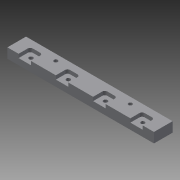
# Autodesk Inventor part: brush rack holder
Saved by Autodesk Inventor 2013 SP2 (Build 170200200, 200)
## iProperties
Created: 2017-05-30
Part Number: brush rack holder
Material: Generic
Document SubType Name: Modeling
Designer: Herman de Vries
Density: 1 g/cm^3
Author: Herman de Vries
Autodesk Inventor part; units mm, degrees
ref_plane "YZ Plane" through (0, 0, 0) normal (1, 0, 0) x (0, 1, 0)
ref_plane "XZ Plane" through (0, 0, 0) normal (0, 1, 0) x (-1, 0, 0)
ref_plane "XY Plane" through (0, 0, 0) normal (0, 0, 1) x (1, 0, 0)
sketch "Sketch1" plane through (0, 0, 0) normal (0, 0, 1) x (1, 0, 0)
  line L0 (0, 0) -> (118, 0)
  line L1 (118, 0) -> (118, 15)
  line L2 (118, 15) -> (0, 15)
  line L3 (0, 15) -> (0, 0)
  dimension "d0" = 118
  dimension "d1" = 15
  constraints: 8 end point, 2 parallel, 1 horizontal, 1 perpendicular
  measures "d0" distance of L2.end L1.end
  measures "d1" distance of L1.end L0.end
extrude "Extrusion1" add sketch "Sketch1" along normal blind 8
sketch "Sketch2" plane through (0, 0, 8) normal (0, 0, 1) x (1, 0, 0)
  circle A0 centre (14, 5) radius 1.6
  circle A1 centre (44, 5) radius 1.6
  circle A2 centre (74, 5) radius 1.6
  line L0 (0, 15) -> (0, 0) projected
  line L1 (118, 0) -> (118, 15) projected
  line L2 (0, 0) -> (118, 0) projected
  circle A3 centre (104, 5) radius 1.5
  line L3 (118, 15) -> (0, 15) projected
  circle A4 centre (29, 10) radius 1.5
  circle A5 centre (89, 10) radius 1.5
  point P0 (59, 0)
  dimension "d4" = 3.2
  dimension "d5" = 3.2
  dimension "d6" = 3.2
  dimension "d11" = 5
  dimension "d14" = 3
  dimension "d15" = 30
  dimension "d16" = 30
  dimension "d17" = 30
  dimension "d18" = 14
  dimension "d19" = 14
  dimension "d20" = 3
  dimension "d21" = 3
  dimension "d22" = 5
  dimension "d23" = 29
  dimension "d24" = 29
  constraints: 6 centre point, 4 horizontal alignment, 1 midpoint
  measures "d4" diameter of A0
  measures "d5" diameter of A1
  measures "d6" diameter of A2
  measures "d11" vertical distance of L0.end A0.centre
  measures "d14" diameter of A3
  measures "d15" distance of A0.centre A1.centre
  measures "d16" distance of A1.centre A2.centre
  measures "d17" distance of A2.centre A3.centre
  measures "d18" distance from line of L1 A3.centre
  measures "d19" distance from line of L0 A0.centre
  measures "d20" diameter of A4
  measures "d21" diameter of A5
  measures "d22" distance from line of L3 A5.centre
  measures "d23" distance from line of L1 A5.centre
  measures "d24" distance from line of L0 A4.centre
extrude "Extrusion2" cut sketch "Sketch2" against normal blind 10 contours A0 | A1 | A2 | A3 | A4 | A5
sketch "Sketch3" plane through (0, 0, 8) normal (0, 0, 1) x (1, 0, 0)
  circle A0 centre (44, 5) radius 1.6 projected
  circle A1 centre (104, 5) radius 1.5 projected
  circle A2 centre (14, 5) radius 1.6 projected
  circle A3 centre (74, 5) radius 1.6 projected
  arc A4 (19, 7.4135) -> (17, 9.4135) centre (17, 7.4135) ccw projected
  line L0 (17, 9.4135) -> (11, 9.4135) projected
  arc A5 (11, 9.4135) -> (9, 7.4135) centre (11, 7.4135) ccw projected
  line L1 (9, 7.4135) -> (9, -0.5865) projected
  arc A6 (19, -0.5865) -> (9, -0.5865) centre (14, -8.0699) ccw projected
  line L2 (19, -0.5865) -> (19, 7.4135) projected
  circle A7 centre (14, 5) radius 1.6 projected
  arc A8 (49, 7.4135) -> (47, 9.4135) centre (47, 7.4135) ccw projected
  line L3 (47, 9.4135) -> (41, 9.4135) projected
  arc A9 (41, 9.4135) -> (39, 7.4135) centre (41, 7.4135) ccw projected
  line L4 (39, 7.4135) -> (39, -0.5865) projected
  arc A10 (49, -0.5865) -> (39, -0.5865) centre (44, -8.0699) ccw projected
  line L5 (49, -0.5865) -> (49, 7.4135) projected
  circle A11 centre (44, 5) radius 1.6 projected
  arc A12 (79, 7.4135) -> (77, 9.4135) centre (77, 7.4135) ccw projected
  line L6 (77, 9.4135) -> (71, 9.4135) projected
  arc A13 (71, 9.4135) -> (69, 7.4135) centre (71, 7.4135) ccw projected
  line L7 (69, 7.4135) -> (69, -0.5865) projected
  arc A14 (79, -0.5865) -> (69, -0.5865) centre (74, -8.0699) ccw projected
  line L8 (79, -0.5865) -> (79, 7.4135) projected
  circle A15 centre (74, 5) radius 1.6 projected
  arc A16 (109, 7.4135) -> (107, 9.4135) centre (107, 7.4135) ccw projected
  line L9 (107, 9.4135) -> (101, 9.4135) projected
  arc A17 (101, 9.4135) -> (99, 7.4135) centre (101, 7.4135) ccw projected
  line L10 (99, 7.4135) -> (99, -0.5865) projected
  arc A18 (109, -0.5865) -> (99, -0.5865) centre (104, -8.0699) ccw projected
  line L11 (109, -0.5865) -> (109, 7.4135) projected
  circle A19 centre (104, 5) radius 1.6 projected
  line L12 (9, -0.5865) -> (19, -0.5865)
  line L13 (39, -0.5865) -> (49, -0.5865)
  line L14 (69, -0.5865) -> (79, -0.5865)
  line L15 (99, -0.5865) -> (109, -0.5865)
  constraints: 8 end point, 3 collinear, 1 perpendicular
extrude "Extrusion3" cut sketch "Sketch3" against normal blind 3 contours A1 | L2 A6 L1 A5 L0 A4 | L12 A6 | L5 A10 L4 A9 L3 A8 | L13 A10 | L8 A14 L7 A13 L6 A12 | L14 A14 | L11 A18 L10 A17 L9 A16 | L15 A18 | A19
equation "\"d15\" = d16"
equation "\"d16\" = d17"
equation "\"d18\" = d19"
equation "\"d23\" = d24"
equation "\"d24\" = d19 + 0.5 * d15"
body "Solid1"
